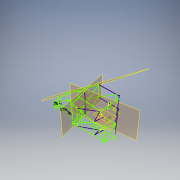
# Autodesk Inventor part: 111
Saved by Autodesk Inventor 2019 (Build 230136000, 136)
## iProperties
Part Number: 111
Material: Genérico
Document SubType Name: Modeling
Designer: João Borges
Density: 1 g/cm^3
Appearance: Padrão
Author: João Borges
Autodesk Inventor part; units mm, degrees
sketch "Assoalho" plane through (0, 0, 0) normal (0, 1, 0) x (-1, 0, 0)
  line L0 (0, 0) -> (0, -310)
  line L1 (-175, 0) -> (-175, -286.2)
  line L2 (-339, 0) -> (-339, -271.128)
  line L3 (-750, -208) -> (0, -310)
  line L4 (0, 0) -> (0, 310)
  line L5 (-175, 0) -> (-175, 286.2)
  line L6 (-339, 0) -> (-339, 271.128)
  line L7 (-750, 208) -> (0, 310)
  line L8 (-750, -208) -> (-750, 208)
  line L9 (0, -310) -> (-750, 208)
  dimension "d5" = 175
  constraints: 20 end point, 2 point on line, 2 vertical
  measures "d5" distance of L0.start L1.start
ref_plane "Plano de trabalho2" through (0, 290, 0) normal (0, 1, 0) x (-1, 0, 0)
sketch "SIM" plane through (0, 290, 0) normal (0, 1, 0) x (-1, 0, 0)
  line L0 (-635.0792, -210.9167) -> (-513.8339, -210.9167) construction
  line L1 (-1143.84, -208) -> (-685.527, -208)
  arc A0 (-592.0818, -237.4632) -> (-685.527, -208) centre (-685.527, -370.9167) ccw
  line L2 (-592.0818, -237.4632) -> (-492.7634, -307.0066)
  arc A1 (-492.7634, -307.0066) -> (-406.5021, -335.3679) centre (-402.6642, -178.3316) ccw
  line L3 (-406.5021, -335.3679) -> (72.8916, -347.0841)
  arc A2 (-685.4637, 215.6215) -> (-591.5206, 246.9682) centre (-688.2017, 380.2696) ccw
  line L4 (-591.5206, 246.9682) -> (-493.3722, 318.1534)
  arc A3 (-408.5522, 347.6124) -> (-493.3722, 318.1534) centre (-402.1758, 192.4142) ccw
  line L5 (-408.5522, 347.6124) -> (70.5804, 367.2979)
  line L6 (-1143.84, 208) -> (-1143.84, -208)
  line L7 (-1143.84, -208) -> (-1143.84, -238)
  line L8 (-1143.84, 208) -> (-1143.84, 238)
  line L9 (-685.4637, 215.6215) -> (-1143.84, 215.6215)
  point P0 (0, 0)
  point P1 (-1243.8402, -210.9167)
  point P2 (-454.8658, -337.1036)
  point P3 (-685.527, -210.9167)
  point P4 (-593.7548, -239.8524)
  point P5 (-1243.8402, 210.003)
  point P6 (-690.8063, 210.003)
  point P7 (-741.2541, 210.003)
  point P8 (-649.4819, 238.9387)
  point P9 (-741.2541, 370.003)
  point P10 (-1243.8402, 212.6709)
  point P11 (-454.8658, 338.8577)
  point P12 (-685.527, 212.6709)
  point P13 (-750, -208)
  point P14 (-1243.8402, -208)
  point P15 (-750, 208)
  point P16 (-1243.8402, 208)
  dimension "d43" = 220
  dimension "d120" = 30
  constraints: 20 end point, 8 point on circle, 4 centre point, 3 vertical, 1 horizontal, 1 perpendicular, 1 point on line
  measures "d43" distance of L0.start point (-454.866, -337.104)
  measures "d120" distance of L6.start L8.end
ref_plane "Plano de trabalho6" through (1243.8402, 290, 0) normal (-0.9506165, 0.3103678, 0) x (0, 0, -1)
ref_plane "Plano de trabalho7" through (750, 0, -208) normal (0.0697565, -0.9975641, 0) x (0, 0, 1)
ref_plane "Plano de trabalho9" through (1243.8402, 290, -210.9167) normal (0.9596242, -0.2812853, 0) x (0, 0, 1)
ref_plane "angulo de ataque" through (1167.3877, 29.1774, -208.0001) normal (0.0693593, -0.9975917, 0) x (0, 0, 1)
sketch3d "FAB SUSP"
ref_plane "plano do tanque" through (-142.3505, 531.2591, -0.3087) normal (0.190809, -0.981627, 0.0005599) x (-0.0001453, 0.0005422, 0.9999998)
ref_plane "plano fire" through (0, 0, 0) normal (0.9816272, 0.190809, 0) x (0, 0, -1)
sketch "Firewall" plane through (0, 0, 0) normal (0.9816272, 0.190809, 0) x (0, 0, -1)
  line L0 (208.0001, 1199.5797) -> (378.6151, 762.8897)
  line L1 (-208.4266, 1199.9999) -> (-377.0246, 770.967)
  arc A0 (388.8009, 688.8354) -> (378.6151, 762.8897) centre (229.5857, 704.6638) ccw
  arc A1 (-377.0246, 770.967) -> (-387.4098, 697.4944) centre (-228.1101, 712.4478) ccw
  line L2 (-373.5449, 549.7904) -> (374.9777, 549.7904)
  line L3 (-340.0001, -0.2101) -> (340.0002, -0.2101)
  line L4 (310.0001, -0.4201) -> (-208.4266, 1199.9999)
  line L5 (-238.4267, 1199.76) -> (237.5731, 1199.76)
  line L6 (-387.4098, 697.4944) -> (-310, 0)
  line L7 (310.0001, -0.4201) -> (388.8009, 688.8354)
  point P0 (0, 0)
  point P1 (-350, 298.9658)
  point P2 (350.0001, 298.5456)
  point P3 (-395, 778.3526)
  point P4 (396.7361, 768.6549)
  dimension "d133" = 160
  dimension "d183" = 549.7904
  constraints: 16 end point, 4 point on circle, 3 horizontal, 2 centre point, 2 coincident, 2 tangent, 1 equal radius
  measures "d133" radius of A0
  measures "d183" distance from line of point (0, 0) L2
sketch "Posição eixo final" plane through (0, 0, 0) normal (0, 0, 1) x (1, 0, 0)
  line L0 (0, 0) -> (-570, 0)
  line L1 (-570, 0) -> (-570, 10)
  circle A0 centre (-570, 10) radius 12.5
  dimension "d188" = 570
  dimension "d189" = 10
  dimension "d190" = 25
  constraints: 4 end point, 1 centre point, 1 coincident, 1 horizontal, 1 perpendicular
  measures "d188" distance of L0.start L0.end
  measures "d189" distance of L0.end L1.end
  measures "d190" diameter of A0
sketch3d "TRASEIRA"
sketch "OSIM" plane through (0, 290, 0) normal (0, 1, 0) x (-1, 0, 0)
  line L0 (-635.0792, -210.9167) -> (-513.8339, -210.9167) construction
  line L1 (0, 0) -> (-92.969, 0)
  line L2 (-1143.84, -208) -> (-790.5859, -208)
  line L3 (-719.9653, -235.2972) -> (-657.1896, -292.3512)
  arc A0 (-657.1896, -292.3512) -> (-591.7716, -319.5194) centre (-586.569, -214.6484) ccw
  line L4 (-1143.84, 208) -> (-790.5859, 208)
  line L5 (-719.9653, 235.2972) -> (-657.1896, 292.3512)
  arc A1 (-790.5859, 208) -> (-719.9653, 235.2972) centre (-790.5859, 313) ccw
  arc A2 (-591.7716, 319.5194) -> (-657.1896, 292.3512) centre (-586.569, 214.6484) ccw
  line L6 (-790.5859, -208) -> (-790.5859, -208)
  arc A3 (-719.9653, -235.2972) -> (-790.5859, -208) centre (-790.5859, -313) ccw
  line L7 (-591.7716, 319.5194) -> (56.424, 342.8186)
  line L8 (-591.7716, -319.5194) -> (56.1351, -343.6827)
  point P0 (-1243.8402, -210.9167)
  point P1 (-649.4819, 238.9387)
  point P2 (-690.8063, 210.003)
  point P3 (-741.2541, 370.003)
  point P4 (-741.2541, 210.003)
  point P5 (-1243.8402, 210.003)
  point P6 (-454.8658, 338.8577)
  point P7 (-685.527, 212.6709)
  point P8 (-1243.8402, 212.6709)
  point P9 (-1243.8402, -208)
  point P10 (-1243.8402, 208)
  point P11 (60.2645, -351.8668)
  point P12 (60.2645, 351.8668)
  dimension "d150" = 105
  constraints: 18 end point, 8 point on circle, 6 symmetric about line, 4 centre point, 4 horizontal, 2 tangent, 1 other
  measures "d150" radius of A3
sketch3d "FAB,FBM,RHO"
sketch "Boneco De M" plane through (0, 0, 0) normal (0, 0, 1) x (1, 0, 0)
  line L0 (100.0575, 119.4039) -> (-125.5508, 886.933)
  line L1 (100.0575, 119.4039) -> (575.1964, 275.1055)
  line L2 (575.1964, 275.1055) -> (1019.3106, 68.0728)
  line L3 (100.0575, 119.4039) -> (-69.1487, 695.0507)
  line L4 (-69.1487, 695.0507) -> (87.7059, 404.7119)
  line L5 (-69.1487, 695.0507) -> (260.8513, 695.0507) construction
  line L6 (87.7059, 404.7119) -> (397.1666, 422.9889)
  arc A0 (-79.7011, 730.9504) -> (-125.5508, 886.933) centre (-81.3953, 815.1823) ccw
  point P0 (0, 0)
  dimension "d169" = 800
  dimension "d170" = 500
  dimension "d171" = 490
  dimension "d172" = 600
  dimension "d175" = 88.236
  dimension "d178" = 330
  dimension "d179" = 61.62
  dimension "d180" = 310
  dimension "d181" = 115
  dimension "d182" = 136.863
  constraints: 14 end point, 2 point on circle, 2 point on line, 1 centre point, 1 equal length, 1 horizontal
  measures "d169" distance of L0.start L0.end
  measures "d170" distance of L0.start L1.end
  measures "d171" distance of L1.end L2.end
  measures "d172" distance of L0.start L3.end
  measures "d175" angle of L1 L0
  measures "d178" distance of L3.end L4.end
  measures "d179" angle of L4 L5
  measures "d180" distance of L4.end L6.end
  measures "d181" angle of L4 L6
  measures "d182" angle of L1 L2
ref_plane "Plano de trabalho15" through (15.4115, 2.9957, 0) normal (0.9816272, 0.190809, 0) x (0, 0, -1)
sketch "Esboço26" plane through (-142.3505, 531.2591, -0.3087) normal (0.190809, -0.981627, 0.0005599) x (-0.0001453, 0.0005422, 0.9999998)
  line L0 (-373.237, -38.3514) -> (-160.541, 418.9921) projected
  line L1 (-305.8589, 106.5265) -> (-160.541, 106.5265)
  line L2 (-160.541, 106.5265) -> (-160.541, -38.3514)
  point P0 (0, -38.3661)
  point P1 (-139.1534, 464.9803)
  constraints: 4 end point, 1 horizontal, 1 perpendicular, 1 point on line
ref_plane "Plano de trabalho16" through (657.1896, 290, -292.3512) normal (0.9965639, 0.0828279, 0) x (-0.0823282, 0.9905518, 0.1096777)
sketch "Esboço27" plane through (657.1896, 290, -292.3512) normal (0.9965639, 0.0828279, 0) x (-0.0823282, 0.9905518, 0.1096777)
  line L0 (769.0814, 0) -> (0, 0) projected
  line L1 (313.7984, 0) -> (438.6359, 0)
  line L2 (438.6359, 0) -> (438.6359, 106.1165)
  line L3 (438.6359, 106.1165) -> (313.7984, 106.1165)
  line L4 (313.7984, 106.1165) -> (313.7984, 0)
  point P0 (-201.0904, 316.3146)
  constraints: 8 end point, 2 parallel, 1 horizontal, 1 perpendicular, 1 point on line
ref_plane "Plano de trabalho18" through (750, 0, 428) normal (-0.0000001, 0.0000002, 1) x (0.9975656, 0.0697345, 0.0000001)
ref_plane "Plano de trabalho17" through (750, 0, 208) normal (-0.0000001, 0.0000002, 1) x (0.9975656, 0.0697345, 0.0000001)
extrude "Extrusão1" add sketch "Esboço27" along normal blind 1.5
sketch3d "Esboço 3D15"
ref_plane "Plano de trabalho19" through (621.7577, 699.6987, 151.4268) normal (-0.99659, -0.0812596, 0.0143283) x (0.0823337, -0.9907596, 0.1077804)
ref_plane "Plano de trabalho20" through (-615.0988, 383.4544, 118.7414) normal (0.5902078, -0.198516, -0.7824616) x (0.4348781, 0.8948063, 0.1010083)
sketch "Esboço28" plane through (-615.0988, 383.4544, 118.7414) normal (0.5902078, -0.198516, -0.7824616) x (0.4348781, 0.8948063, 0.1010083)
  line L0 (886.3239, 1.5116) -> (836.3239, 1.5116)
  line L1 (886.3239, 1.5116) -> (850.9686, 36.8669)
  line L2 (850.9686, 36.8669) -> (836.3239, 1.5116)
  point P0 (-87.6183, 498.7078)
  dimension "d245" = 50
  dimension "d246" = 50
  constraints: 6 end point, 1 horizontal
  measures "d245" distance of L0.start L0.end
  measures "d246" distance of L0.start L1.end
extrude "Extrusão2" add sketch "Esboço28" along normal blind 1.5
